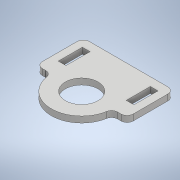
# Autodesk Inventor part: Гор. шарнир
Saved by Autodesk Inventor 2020 (Build 240168000, 168)
## iProperties
Created: 2020-02-22
Part Number: Гор. шарнир
Material: Типовые
Document SubType Name: Modeling
Designer: Leancher
Density: 1 g/cm^3
Appearance: По умолчанию
Author: Leancher
Autodesk Inventor part; units mm, degrees
ref_plane "YZ Plane" through (0, 0, 0) normal (1, 0, 0) x (0, 1, 0)
ref_plane "XZ Plane" through (0, 0, 0) normal (0, 1, 0) x (-1, 0, 0)
ref_plane "XY Plane" through (0, 0, 0) normal (0, 0, 1) x (1, 0, 0)
sketch "Эскиз1" plane through (0, 0, 0) normal (0, 0, 1) x (1, 0, 0)
  line L0 (32.4057, 38.6485) -> (-32.4072, 38.6485)
  arc A0 (-32.4072, 38.6485) -> (-37.4072, 33.6485) centre (-32.4072, 33.6485) ccw
  line L1 (-37.4072, 33.6485) -> (-37.4072, 5)
  arc A1 (-37.4072, 5) -> (-32.4072, 0) centre (-32.4072, 5) ccw
  line L2 (-30, 0) -> (-29.5804, 0)
  arc A2 (-24.6503, -4.1667) -> (-29.5804, 0) centre (-29.5804, -5) ccw
  arc A3 (-24.6503, -4.1667) -> (24.6503, -4.1667) centre (0, 0) ccw
  arc A4 (29.5804, 0) -> (24.6503, -4.1667) centre (29.5804, -5) ccw
  circle A5 centre (0, 0) radius 13.45
  line L3 (-0.0007, 35) -> (-0.0007, -40.0249) construction
  line L4 (-31.1692, 11.8598) -> (-24.8192, 11.8598)
  line L5 (-24.8192, 11.8598) -> (-24.8192, 31.7098)
  line L6 (-24.8192, 31.7098) -> (-31.1692, 31.7098)
  line L7 (-31.1692, 31.7098) -> (-31.1692, 11.8598)
  line L8 (24.8177, 11.8598) -> (31.1677, 11.8598)
  line L9 (31.1677, 11.8598) -> (31.1677, 31.7098)
  line L10 (31.1677, 31.7098) -> (24.8177, 31.7098)
  line L11 (24.8177, 31.7098) -> (24.8177, 11.8598)
  arc A6 (37.4057, 33.6485) -> (32.4057, 38.6485) centre (32.4057, 33.6485) ccw
  line L12 (37.4057, 33.6485) -> (37.4057, 5)
  arc A7 (32.4057, 0) -> (37.4057, 5) centre (32.4057, 5) ccw
  line L13 (32.4057, 0) -> (29.5804, 0)
  line L14 (-32.4072, 0) -> (-30, 0)
  point P0 (29.9986, 30)
  point P1 (-30, 30)
  point P2 (25.9869, 30)
  constraints: 30 end point, 15 point on circle, 8 centre point, 6 symmetric about line, 1 collinear, 1 horizontal, 1 tangent, 1 vertical, 2 other
extrude "Выдавливание1" add sketch "Эскиз1" along normal blind 5
